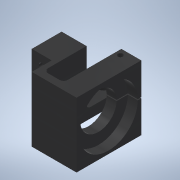
# Autodesk Inventor part: pulley_positioner
Saved by Autodesk Inventor 2021 (Build 250183000, 183)
## iProperties
Created: 2022-04-14
Part Number: pulley_positioner
Material: ABS Plastic
Document SubType Name: Modeling
Designer: 10154704
Density: 1.06 g/cm^3
Appearance: Dark Gray
Author: 10154704
Autodesk Inventor part; units mm, degrees
ref_plane "YZ Plane" through (0, 0, 0) normal (1, 0, 0) x (0, 1, 0)
ref_plane "XZ Plane" through (0, 0, 0) normal (0, 1, 0) x (-1, 0, 0)
ref_plane "XY Plane" through (0, 0, 0) normal (0, 0, 1) x (1, 0, 0)
sketch "Skizze1" plane through (0, 0, 0) normal (0, 0, 1) x (1, 0, 0)
  line L0 (0, 20) -> (0, 50)
  line L1 (0, 50) -> (25, 50)
  line L2 (65, 0) -> (20, 0)
  line L3 (20, 0) -> (20, 20)
  line L4 (20, 20) -> (0, 20)
  line L5 (25, 50) -> (25, 7)
  line L6 (25, 7) -> (45, 7)
  line L7 (45, 7) -> (45, 65)
  line L8 (45, 65) -> (65, 65)
  line L9 (65, 65) -> (65, 0)
  point P0 (0, 0)
  dimension "d2" = 20
  dimension "d3" = 20
  dimension "d8" = 20
  dimension "d10" = 7
  dimension "d11" = 5
  dimension "d18" = 50
  dimension "d44" = 20
  dimension "d69" = 65
  constraints: 20 end point, 7 perpendicular, 2 point on line, 2 vertical, 1 horizontal
  measures "d2" distance from line of point (0, 0) L4
  measures "d3" distance from line of point (0, 0) L3
  measures "d8" distance between parallel lines of L7 L5
  measures "d10" distance between parallel lines of L2 L6
  measures "d11" distance between parallel lines of L5 L3
  measures "d18" distance between parallel lines of L2 L1
  measures "d44" distance between parallel lines of L9 L7
  measures "d69" distance between parallel lines of L8 L2
extrude "Extrusion1" add sketch "Skizze1" along normal blind 65
ref_plane "Arbeitsebene1" through (35, 7, 0) normal (1, 0, 0) x (0, 0, -1)
sketch "Skizze5" plane through (0, 50, 0) normal (0, 1, 0) x (1, 0, 0)
  line L0 (0, 0) -> (0, -65) projected
  line L1 (0, 0) -> (25, 0) projected
  line L2 (25, -65) -> (0, -65) projected
  point P0 (10, -22)
  point P1 (10, -55)
  dimension "d32" = 10
  dimension "d33" = 10
  dimension "d34" = 22
  dimension "d35" = 10
  measures "d32" distance from line of point (10, -22) L0
  measures "d33" distance from line of L0 point (10, -55)
  measures "d34" distance from line of L1 point (10, -22)
  measures "d35" distance from line of L2 point (10, -55)
hole "Bohrung2" at (10, 50, 55) at (10, 50, 22) direction (0, -1, 0) diameter 5.5 end up to face face through (13.3333, 20, 21.6667) facing (0, -1, 0) counterbore diameter 9 counterbore depth 5
sketch "Skizze8" plane through (0, 0, 0) normal (0, 0, 1) x (1, 0, 0)
  line L0 (0, 20) -> (0, 50) projected
  line L1 (0, 50) -> (25, 50) projected
  line L2 (25, 50) -> (25, 7) projected
  line L3 (25, 7) -> (45, 7) projected
  line L4 (45, 7) -> (45, 65) projected
  line L5 (45, 65) -> (65, 65) projected
  line L6 (65, 65) -> (65, 0) projected
  line L7 (65, 0) -> (20, 0) projected
  line L8 (20, 0) -> (20, 20) projected
  line L9 (20, 20) -> (0, 20) projected
  line L10 (25, 50) -> (0, 50) projected
  line L11 (0, 50) -> (25, 50)
  line L12 (25, 50) -> (25, 92)
  line L13 (25, 92) -> (0, 92)
  line L14 (0, 92) -> (0, 50)
  line L15 (25, 7) -> (25, 50) projected
  point P0 (0, 0)
  dimension "d102" = 42
  constraints: 8 end point, 2 parallel, 1 collinear, 1 horizontal, 1 perpendicular
  measures "d102" distance between parallel lines of L1 L13
extrude "Extrusion6" add sketch "Skizze8" along normal blind 10 contours L14 L13 L12 L1
sketch "Skizze9" plane through (0, 0, 10) normal (0, 0, 1) x (1, 0, 0)
  line L0 (0, 20) -> (20, 20) projected
  line L1 (25, 92) -> (0, 92) projected
  line L2 (25, 50) -> (0, 50) projected
  point P0 (0, 0)
  point P1 (12.5, 80)
  dimension "d61" = 20
  dimension "d62" = 12.5
  dimension "d70" = 25
  dimension "d71" = 30
  measures "d61" distance of L0.start L0.end
  measures "d62" horizontal distance of L0.start point (12.5, 80)
  measures "d70" distance of L1.start L1.end
  measures "d71" distance from line of L2 point (12.5, 80)
hole "Bohrung3" at (12.5, 80, 10) direction (0, 0, -1) diameter 14 end up to face face through (8.3333, 68, 0) facing (0, 0, -1)
sketch "Skizze10" plane through (65, 0, 0) normal (1, 0, 0) x (0, 0, -1)
  line L0 (0, 0) -> (-65, 0) projected
  circle A0 centre (-32.5, 32) radius 18.25
  dimension "d63" = 65
  dimension "d64" = 32.5
  dimension "d65" = 36.5
  dimension "d66" = 32
  constraints: 1 centre point
  measures "d63" distance of L0.start L0.end
  measures "d64" horizontal distance of A0.centre L0.end
  measures "d65" diameter of A0
  measures "d66" distance from line of L0 A0.centre
extrude "Extrusion7" cut sketch "Skizze10" against normal up to surface (20 mm away)
sketch "Skizze11" plane through (65, 0, 0) normal (1, 0, 0) x (0, 0, -1)
  line L0 (-33, 65) -> (-32, 65)
  line L1 (-32, 65) -> (-32, 32)
  line L2 (-32, 32) -> (-33, 32)
  line L3 (-33, 32) -> (-33, 65)
  circle A0 centre (-32.5, 32) radius 18.25 projected
  line L4 (0, 65) -> (-65, 65) projected
  point P0 (0, 0)
  dimension "d72" = 1
  dimension "d73" = 0.5
  constraints: 8 end point, 2 parallel, 1 collinear, 1 horizontal, 1 midpoint, 1 perpendicular
  measures "d72" distance between parallel lines of L1 L3
  measures "d73" distance from line of L3 A0.centre
extrude "Extrusion8" cut sketch "Skizze11" against normal up to surface (20 mm away) contours L0 L1 A0 L3 | A0 L1 L2 L3 picked at (-32.4444, 38.0831)
sketch "Skizze12" plane through (0, 0, 65) normal (0, 0, 1) x (1, 0, 0)
  line L0 (65, 65) -> (45, 65) projected
  line L1 (65, 50.2431) -> (45, 50.2431) projected
  line L2 (45, 65) -> (45, 7) projected
  point P0 (0, 0)
  point P1 (50, 59)
  dimension "d76" = 20
  dimension "d78" = 6
  dimension "d90" = 5
  measures "d76" distance of L0.start L0.end
  measures "d78" distance from line of L0 point (50, 59)
  measures "d90" distance from line of L2 point (50, 59)
hole "Bohrung4" at (50, 59, 65) direction (0, 0, -1) diameter 5 end up to face face through (58.3333, 24, 0) facing (0, 0, -1)
fillet "Rundung2" radius 4 5 edges at (0, 92, 5) (25, 92, 5) (12.5, 50, 10) (25, 7, 32.5) (45, 7, 32.5)
sketch "Skizze13" plane through (65, 0, 0) normal (1, 0, 0) x (0, 0, -1)
  arc A0 (-33, 50.2431) -> (-32, 50.2431) centre (-32.5, 32) ccw projected
  circle A1 centre (-32.5, 32) radius 29.5
  point P0 (0, 0)
  dimension "d87" = 59
  constraints: 1 centre point, 1 coincident
  measures "d87" diameter of A1
extrude "Extrusion9" cut sketch "Skizze13" against normal blind 10
sketch "Skizze14" plane through (0, 0, 65) normal (0, 0, 1) x (1, 0, 0)
  circle A0 centre (50, 59) radius 2.5 projected
  line L0 (0, 50) -> (0, 20) projected
  line L1 (0, 20) -> (20, 20) projected
  line L2 (20, 20) -> (20, 0) projected
  line L3 (20, 0) -> (65, 0) projected
  line L4 (65, 0) -> (65, 65) projected
  line L5 (65, 65) -> (45, 65) projected
  line L6 (45, 65) -> (45, 11) projected
  arc A1 (41, 7) -> (45, 11) centre (41, 11) ccw projected
  line L7 (41, 7) -> (29, 7) projected
  arc A2 (25, 11) -> (29, 7) centre (29, 11) ccw projected
  line L8 (25, 11) -> (25, 50) projected
  line L9 (25, 50) -> (0, 50) projected
  line L10 (65, 61.4958) -> (65, 2.5) projected
  line L11 (55, 61.4958) -> (65, 61.4958) projected
  line L12 (55, 61.4958) -> (55, 61.4958) projected
  line L13 (65, 61.4958) -> (55, 61.4958) projected
  line L14 (65, 61.4958) -> (65, 61.4958) projected
  line L15 (65, 2.5) -> (55, 2.5) projected
  point P0 (0, 0)
  point P1 (59, 31.9979)
  dimension "d92" = 58.9958
  dimension "d93" = 29.4979
  dimension "d94" = 6
  measures "d92" distance between parallel lines of L15 L13
  measures "d93" distance from line of L15 point (59, 31.998)
  measures "d94" distance from line of L4 point (59, 31.998)
hole "Bohrung5" [suppressed]
equation "\"d2\" = b"
equation "\"d3\" = b"
equation "\"d32\" = 0.5 * b"
equation "\"d33\" = d32"
equation "\"d62\" = 0.5 * d70"
equation "\"d64\" = 0.5 * d63"
equation "\"d73\" = 0.5 * d72"
equation "\"d93\" = 0.5 * d92"
equation "\"b\" = 20"
